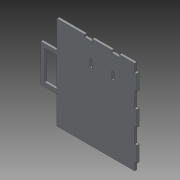
# Autodesk Inventor part: Mid Plate
Saved by Autodesk Inventor 2015 (Build 190159000, 159)
## iProperties
Created: 2014-07-26
Part Number: Mid Plate
Material: Generic
Document SubType Name: Modeling
Designer: karl
Density: 1 g/cm^3
Appearance: Default
Author: karl
Autodesk Inventor part; units mm, degrees
ref_plane "YZ Plane" through (0, 0, 0) normal (1, 0, 0) x (0, 1, 0)
ref_plane "XZ Plane" through (0, 0, 0) normal (0, 1, 0) x (-1, 0, 0)
ref_plane "XY Plane" through (0, 0, 0) normal (0, 0, 1) x (1, 0, 0)
sketch "Sketch1" plane through (0, 0, 0) normal (0, 1, 0) x (-1, 0, 0)
  line L0 (50, 60) -> (-50, 60)
  line L1 (-50, 60) -> (-50, -60)
  line L2 (-50, -60) -> (50, -60)
  line L3 (50, -60) -> (50, 60)
  line L4 (50, 60) -> (-50, -60) construction
  line L5 (-50, 60) -> (50, -60) construction
  point P0 (0, 0)
  dimension "d0" = 60
  dimension "d1" = 100
  constraints: 12 end point, 2 midpoint, 2 parallel, 1 horizontal, 1 perpendicular
  measures "d0" distance from line of L2 point (0, 0)
  measures "d1" distance between parallel lines of L3 L1
extrude "Extrusion1" add sketch "Sketch1" along normal blind 3
sketch "Sketch2" plane through (0, 3, 0) normal (0, 1, 0) x (1, 0, 0)
  line L0 (-50, -60) -> (50, -60) projected
  line L1 (-14.5, -60) -> (-4.5, -60)
  line L2 (-4.5, -60) -> (-4.5, -57)
  line L3 (-4.5, -57) -> (-14.5, -57)
  line L4 (-14.5, -57) -> (-14.5, -60)
  line L5 (50, -60) -> (50, 60) projected
  line L6 (20.5, -60) -> (30.5, -60)
  line L7 (30.5, -60) -> (30.5, -57)
  line L8 (30.5, -57) -> (20.5, -57)
  line L9 (20.5, -57) -> (20.5, -60)
  line L10 (-4.5, -37) -> (-7.5, -37)
  line L11 (-7.5, -37) -> (-7.5, -27)
  line L12 (-7.5, -27) -> (-4.5, -27)
  line L13 (-4.5, -27) -> (-4.5, -37)
  line L14 (20.5, -27) -> (23.5, -27)
  line L15 (23.5, -27) -> (23.5, -37)
  line L16 (23.5, -37) -> (20.5, -37)
  line L17 (20.5, -37) -> (20.5, -27)
  point P0 (0, 0)
  dimension "d4" = 10
  dimension "d5" = 3
  dimension "d6" = 54.5
  dimension "d7" = 10
  dimension "d8" = 3
  dimension "d9" = 25
  dimension "d10" = 3
  dimension "d11" = 10
  dimension "d12" = 30
  dimension "d13" = 3
  dimension "d14" = 10
  constraints: 32 end point, 8 parallel, 4 horizontal, 4 perpendicular, 3 collinear, 2 point on line
  measures "d4" distance of L3.end L2.end
  measures "d5" distance of L2.end L1.end
  measures "d6" distance between parallel lines of L5 L2
  measures "d7" distance of L8.end L7.end
  measures "d8" distance of L7.end L6.end
  measures "d9" distance between parallel lines of L2 L9
  measures "d10" distance of L11.end L12.end
  measures "d11" distance of L10.end L11.end
  measures "d12" distance between parallel lines of L3 L12
  measures "d13" distance of L15.end L16.end
  measures "d14" distance of L14.end L15.end
extrude "Extrusion2" cut sketch "Sketch2" against normal blind 3
sketch "Sketch3" plane through (0, 3, 0) normal (0, 1, 0) x (1, 0, 0)
  line L0 (50, -60) -> (50, 60) projected
  line L1 (50, 10) -> (53, 10)
  line L2 (53, 10) -> (53, -10)
  line L3 (53, -10) -> (50, -10)
  line L4 (50, -10) -> (50, 10)
  line L5 (50, -30) -> (53, -30)
  line L6 (53, -30) -> (53, -50)
  line L7 (53, -50) -> (50, -50)
  line L8 (50, -50) -> (50, -30)
  line L9 (50, 30) -> (53, 30)
  line L10 (53, 30) -> (53, 50)
  line L11 (53, 50) -> (50, 50)
  line L12 (50, 50) -> (50, 30)
  point P0 (0, 0)
  point P1 (53, 0)
  dimension "d17" = 3
  dimension "d18" = 20
  dimension "d19" = 3
  dimension "d20" = 20
  dimension "d21" = 20
  dimension "d22" = 20
  constraints: 24 end point, 6 parallel, 3 horizontal, 3 perpendicular, 3 point on line, 2 collinear, 1 horizontal alignment, 1 midpoint
  measures "d17" distance of L2.end L3.end
  measures "d18" distance of L1.end L2.end
  measures "d19" distance of L6.end L7.end
  measures "d20" distance of L5.end L6.end
  measures "d21" distance between parallel lines of L3 L5
  measures "d22" distance between parallel lines of L1 L9
extrude "Extrusion3" add sketch "Sketch3" against normal blind 3
sketch "Sketch4" plane through (0, 3, 0) normal (0, 1, 0) x (1, 0, 0)
  line L0 (-50, 60) -> (-50, -60) projected
  line L1 (-50, 24) -> (-71, 24)
  line L2 (-71, 24) -> (-71, -24)
  line L3 (-71, -24) -> (-50, -24)
  line L4 (-50, -24) -> (-50, 24)
  line L5 (-50, -19) -> (-66, -19)
  line L6 (-66, -19) -> (-66, 19)
  line L7 (-66, 19) -> (-50, 19)
  line L8 (-50, 19) -> (-50, -19)
  point P0 (0, 0)
  point P1 (-71, 0)
  point P2 (-66, 0)
  dimension "d27" = 38
  dimension "d28" = 16
  dimension "d29" = 5
  dimension "d30" = 5
  constraints: 16 end point, 4 parallel, 2 horizontal, 2 horizontal alignment, 2 midpoint, 2 perpendicular, 2 point on line
  measures "d27" distance of L5.end L6.end
  measures "d28" distance of L5.start L5.end
  measures "d29" distance between parallel lines of L1 L7
  measures "d30" distance between parallel lines of L6 L2
extrude "Extrusion4" add sketch "Sketch4" against normal blind 3 contours L0 L7 L6 L5 L3 L2 L1
sketch "Sketch6" plane through (0, 3, 0) normal (0, 1, 0) x (1, 0, 0)
  line L0 (-50, 60) -> (-50, 24) projected
  line L1 (-50, 47) -> (-53, 47)
  line L2 (-53, 47) -> (-53, 37)
  line L3 (-53, 37) -> (-50, 37)
  line L4 (-50, 37) -> (-50, 47)
  line L5 (-50, 24) -> (-71, 24) projected
  point P0 (0, 0)
  dimension "d39" = 3
  dimension "d40" = 10
  dimension "d41" = 13
  dimension "d42" = 13
  constraints: 8 end point, 2 parallel, 1 horizontal, 1 perpendicular, 1 point on line
  measures "d39" distance of L3.end L2.end
  measures "d40" distance of L2.end L1.end
  measures "d41" distance from line of L0.start L1
  measures "d42" distance between parallel lines of L5 L3
extrude "Extrusion6" add sketch "Sketch6" against normal blind 3
sketch "Sketch8" plane through (0, 3, 0) normal (0, 1, 0) x (1, 0, 0)
  line L0 (20.5, -37) -> (-4.5, -37)
  line L1 (-4.5, -37) -> (-4.5, 37)
  line L2 (-4.5, 37) -> (20.5, 37)
  line L3 (20.5, 37) -> (20.5, -37)
  line L4 (-4.5, -27) -> (-4.5, -37) projected
  point P0 (0, 0)
  point P1 (20.5, 0)
  constraints: 8 end point, 2 parallel, 1 collinear, 1 horizontal, 1 horizontal alignment, 1 midpoint, 1 perpendicular
extrude "Extrusion7" cut sketch "Sketch8" against normal blind 3
mirror "Mirror1" about plane through (0, 0, 0) normal (0, 0, 1) of "Extrusion2"
mirror "Mirror2" about plane through (0, 0, 0) normal (0, 0, 1) of "Extrusion6"
equation "\"d30\" = d29"
equation "\"d41\" = d42"
body "Solid1"
